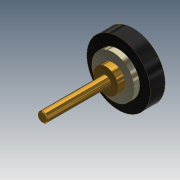
# Autodesk Inventor part: Вал последний с чем то
Saved by Autodesk Inventor 2017 (Build 210142000, 142)
## iProperties
Created: 2018-08-24
Part Number: Вал последний с чем то
Material: Латунь, мягкая, желтая
Document SubType Name: Modeling
Designer: Shepelev
Density: 8.47 g/cm^3
Appearance: Латунь - сатинированная
Author: Shepelev
Autodesk Inventor part; units mm, degrees
ref_plane "YZ Plane" through (0, 0, 0) normal (1, 0, 0) x (0, 1, 0)
ref_plane "XZ Plane" through (0, 0, 0) normal (0, 1, 0) x (-1, 0, 0)
ref_plane "XY Plane" through (0, 0, 0) normal (0, 0, 1) x (1, 0, 0)
sketch "Эскиз1" plane through (0, 0, 0) normal (1, 0, 0) x (0, 1, 0)
  line L0 (0, 13.5) -> (0.7, 13.5)
  line L1 (0.7, 13.5) -> (0.7, 4.5)
  line L2 (0.7, 4.5) -> (1.75, 4.5)
  line L3 (1.75, 4.5) -> (1.75, 3.5)
  line L4 (1.75, 3.5) -> (3, 3.5)
  line L5 (3, 3.5) -> (3, 2.7)
  line L6 (3, 2.7) -> (4.5, 2.7)
  line L7 (4.5, 2.7) -> (4.5, 0.6)
  line L8 (0, 0) -> (0, 13.5)
  line L9 (1.6477, 0.4) -> (1, 0.4)
  line L10 (1, 0.4) -> (1, 0)
  line L11 (1, 0) -> (0, 0)
  line L12 (0, -2.7) -> (0, 16.2) projected
  line L13 (4.5, 0.6) -> (1.6477, 0.6)
  line L14 (1.6477, 0.6) -> (1.6477, 0.4)
  dimension "d0" = 1.4
  dimension "d1" = 13.5
  dimension "d2" = 9
  dimension "d3" = 2
  dimension "d4" = 0.4
  dimension "d5" = 0.2
  dimension "d6" = 9
  dimension "d7" = 1
  dimension "d8" = 0.8
  dimension "d9" = 3.5
  dimension "d10" = 6
  constraints: 28 end point, 10 perpendicular, 3 horizontal, 1 point on line
  measures "d0" diameter of L1 L12
  measures "d1" distance of L8.start L0.start
  measures "d2" diameter of L7 L12
  measures "d3" diameter of L10 L12
  measures "d4" distance of L9.end L10.end
  measures "d5" distance between parallel lines of L9 L13
  measures "d6" distance of L0.end L1.end
  measures "d7" distance of L2.end L3.end
  measures "d8" distance of L4.end L5.end
  measures "d9" diameter of L3 L12
  measures "d10" diameter of L5 L12
revolve "Вращение1" add sketch "Эскиз1" angle 360 about axis through (0, 0, -10) along (0, 0, 1)
chamfer "Фаска1" distance 0.1 angle 45 1 edges at (0, -0.7, 13.5)
